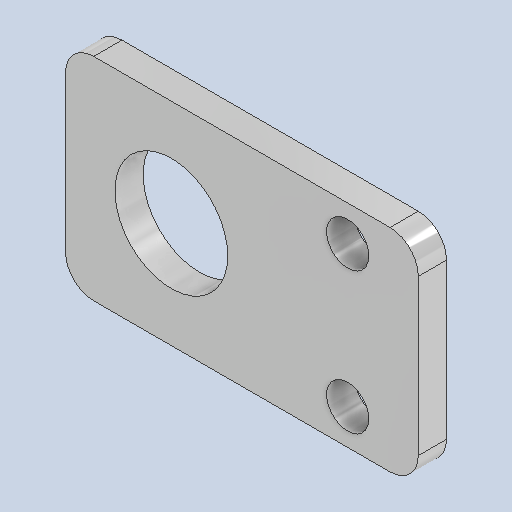
# Autodesk Inventor part: finger_al_mk_1
Saved by Autodesk Inventor 2024.1 (Build 281209000, 209)
## iProperties
Created: 2022-06-23
Part Number: finger_al_mk_1
Material: アルミニウム 6061-AHC
Document SubType Name: Modeling
Designer: zegi
Density: 2.7 g/cm^3
Appearance: アルミニウム - ダーク
Mass: 1.65868 g
Surface Area: 8.55425 cm^2
Volume: 0.614327 cm^3
Author: zegi
Autodesk Inventor part; units mm, degrees
ref_plane "YZ Plane" through (0, 0, 0) normal (1, 0, 0) x (0, 1, 0)
ref_plane "XZ Plane" through (0, 0, 0) normal (0, 1, 0) x (-1, 0, 0)
ref_plane "XY Plane" through (0, 0, 0) normal (0, 0, 1) x (1, 0, 0)
sketch "スケッチ1" plane through (0, 0, 0) normal (0, 0, 1) x (1, 0, 0)
  line L0 (0, 0) -> (15, 0)
  line L1 (15, 0) -> (15, 15)
  line L2 (15, 15) -> (0, 15)
  line L3 (0, 15) -> (0, 0)
  circle A0 centre (7.5, 7.5) radius 4
  line L4 (15, 15) -> (25, 15)
  line L5 (25, 15) -> (25, 0)
  line L6 (25, 0) -> (15, 0)
  line L7 (15, 0) -> (15, 15)
  circle A1 centre (20, 12.5) radius 1.5
  circle A2 centre (20, 2.5) radius 1.5
  dimension "d0" = 15
  dimension "d1" = 15
  dimension "d2" = 8
  dimension "d3" = 7.5
  dimension "d4" = 7.5
  dimension "d5" = 10
  dimension "d6" = 10
  dimension "d7" = 2.5
  dimension "d8" = 2.5
  dimension "d9" = 3
  dimension "d10" = 3
  constraints: 16 end point, 4 parallel, 3 centre point, 3 coincident, 2 horizontal, 2 perpendicular
  measures "d0" distance of L2.end L1.end
  measures "d1" distance of L1.end L0.end
  measures "d2" diameter of A0
  measures "d3" distance from line of point (7.5, 7.5) L2
  measures "d4" distance from line of L3 A0.centre
  measures "d5" distance of L5.end L6.end
  measures "d6" distance of point (20, 2.5) point (20, 12.5)
  measures "d7" distance from line of L4 point (20, 12.5)
  measures "d8" distance from line of L6 point (20, 2.5)
  measures "d9" diameter of A1
  measures "d10" diameter of A2
extrude "押し出し1" add sketch "スケッチ1" along normal blind 2
fillet "フィレット1" radius 2 4 edges at (0, 15, 1) (0, 0, 1) (25, 0, 1) (25, 15, 1)
equation "\"d1\" = d0"
equation "\"d3\" = 0.5 * d0"
equation "\"d4\" = 0.5 * d1"
